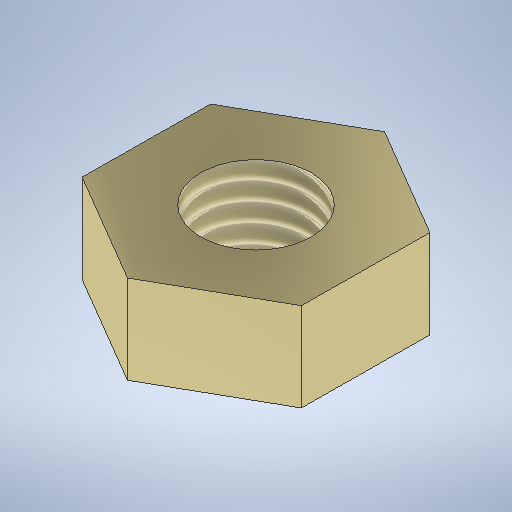
# Autodesk Inventor part: M3 Mutter
Saved by Autodesk Inventor 2025.1 (Build 291241000, 241)
## iProperties
Created: 2024-12-19
Part Number: M3 Mutter
Material: Generisch
Document SubType Name: Modeling
Designer: Julian
Density: 1 g/cm^3
Appearance: Vorgabe
Author: Julian
Autodesk Inventor part; units mm, degrees
ref_plane "YZ Plane" through (0, 0, 0) normal (1, 0, 0) x (0, 1, 0)
ref_plane "XZ Plane" through (0, 0, 0) normal (0, 1, 0) x (-1, 0, 0)
ref_plane "XY Plane" through (0, 0, 0) normal (0, 0, 1) x (1, 0, 0)
sketch "Skizze1" plane through (0, 0, 0) normal (0, 0, 1) x (1, 0, 0)
  line L0 (-2.9798, 1.7507) -> (0.0263, 3.4559)
  line L1 (0.0263, 3.4559) -> (3.0061, 1.7052)
  line L2 (3.0061, 1.7052) -> (2.9798, -1.7507)
  line L3 (2.9798, -1.7507) -> (-0.0263, -3.4559)
  line L4 (-0.0263, -3.4559) -> (-3.0061, -1.7052)
  line L5 (-3.0061, -1.7052) -> (-2.9798, 1.7507)
  point P0 (0, 0)
  constraints: 12 end point, 13 other
extrude "Extrusion1" add sketch "Skizze1" along normal blind 2.4
sketch "Skizze2" plane through (0, 0, 2.4) normal (0, 0, 1) x (1, 0, 0)
  circle A0 centre (0, 0) radius 1.5
  dimension "d3" = 3
  constraints: 1 centre point, 1 coincident
  measures "d3" diameter of A0
extrude "Extrusion2" cut sketch "Skizze2" against normal through all
thread "Gewinde1" size "M3x0.5" class "6H" standard "ANSI Metric M Profile" full length
